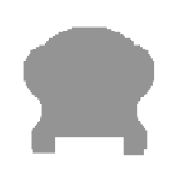
# Autodesk Inventor part: Поручень
Saved by Autodesk Inventor 2019 (Build 230136000, 136)
## iProperties
_CCFamilyDisplayName: Поручень - Ограждение
_FrameMemberDoc: Frame Member File
_Version: 15.0.0
_GetPNFromCC: 1
Created: 2018-10-11
Part Number: Поручень
Material: Древесина (дуб)
Description: Ограждение
Document SubType Name: Modeling
Standard: Без имени
Designer: Андреев Н.Л.
Language: ru-RU
Size Designation: Поручень x75 x58
Categories: <MemberInstance><Categories><Category DisplayName="Профили фасонные" InternalName="089c4875-fa83-4c05-b084-43b9cc11f5ed" Mnemonic="GRDR"><CategoryParameter DisplayName="Вес погонного метра" InternalName="0bb95a10-148f-4027-a459-38d7b056702a" Mnemonic="shpmass"/><CategoryParameter DisplayName="Площадь сечения" InternalName="1ff91680-64b0-4202-b9a3-7fd3f94bba3b" Mnemonic="secarea"/><CategoryParameter DisplayName="Радиус инерции (x)" InternalName="25778675-03e9-40c1-b6a8-4a9ed693320d" Mnemonic="gyrradx"/><CategoryParameter DisplayName="Модуль жесткости при кручении" InternalName="26c1ec35-5026-4c63-ad0a-751cf684a536" Mnemonic="torrigmod"/><CategoryParameter DisplayName="Расстояние центра тяжести X-X" InternalName="26c9bdb8-9c79-4b4f-a92e-8e197583c9c4" Mnemonic="grcendistX"/><CategoryParameter DisplayName="Старое обозначение элемента" InternalName="340afe4f-75d7-48d3-ab7d-943f3c3da468" Mnemonic="LegacyMemberID"/><CategoryParameter DisplayName="Основная длина" InternalName="42e34263-8f20-4d0e-ad48-bf1385b87c24" Mnemonic="shplen"/><CategoryParameter DisplayName="Момент инерции (y)" InternalName="4b9f58ea-bced-460e-81ea-3d29ca5a49e3" Mnemonic="inermomy"/><CategoryParameter DisplayName="Момент инерции (x)" InternalName="4cd780bc-73d7-43ac-917a-579e5cbd684d" Mnemonic="inermomx"/><CategoryParameter DisplayName="Настраиваемые базовые точки" InternalName="4f1d1b73-316d-484b-a3df-9cbabb16eb77" Mnemonic="shpBasePoint"/><CategoryParameter DisplayName="Высота фигуры" InternalName="50274e7d-5ac0-4796-92cb-c59e54983c67" Mnemonic="shpheig"/><CategoryParameter DisplayName="Момент сопротивления сечения (y)" InternalName="59eaa5e9-d227-48dc-b6c1-6920f96e0f95" Mnemonic="secmody"/><CategoryParameter DisplayName="Обозначение разреза" InternalName="5a64d034-428d-49c8-ba32-7619764de20f" Mnemonic="shpdes"/><CategoryParameter DisplayName="Момент сопротивления сечения (x)" InternalName="72cfad18-cf51-4ed4-aaa7-c6b224f8419f" Mnemonic="secmodx"/><CategoryParameter DisplayName="Торсионный момент сопротивления сечения" InternalName="7c55a8dc-8844-49f9-a867-cc677b30ec9a" Mnemonic="torsecmod"/><CategoryParameter DisplayName="Ширина фигуры" InternalName="7c717d54-a18f-4666-b4d4-573cce22c62c" Mnemonic="shpwdth"/><CategoryParameter DisplayName="Толщина второй фигуры" InternalName="9251a8e1-85fd-4e47-af99-afdb762317d9" Mnemonic="shpthick2"/><CategoryParameter DisplayName="Созданные с помощью генератора рам" InternalName="9c666724-f362-4ea7-ac62-f6a007de5c69" Mnemonic="shpFGAuto"/><CategoryParameter DisplayName="Расстояние центра тяжести Y-Y" InternalName="bcc4fb17-7af4-436a-8f8c-d0aa3b0248c5" Mnemonic="grcendistY"/><CategoryParameter DisplayName="Радиус инерции (y)" InternalName="bfa18ebe-1636-4dbe-8d42-b263e0b73184" Mnemonic="gyrrady"/><CategoryParameter DisplayName="Толщина фигуры" InternalName="d109cf76-8eb4-42fc-9800-4409734adc67" Mnemonic="shpthick"/><CategoryParameter DisplayName="Коэффициент смещения при сдвиге" InternalName="de4c90c6-aaa8-468f-a335-6737b311b5d3" Mnemonic="shdispc"/><Category DisplayName="Специальные" InternalName="f02205ff-2390-476f-921c-0b3185f88e84" Mnemonic="OTHSHP"><CategoryParameter DisplayName="Момент инерции (y)" InternalName="044c654e-f649-48ac-84cc-650a29ae31ca" Mnemonic="inermomy"/><CategoryParameter DisplayName="Толщина фигуры" InternalName="12b1a788-9233-48fd-a933-2df8ff42b15f" Mnemonic="shpthick"/><CategoryParameter DisplayName="Вес погонного метра" InternalName="2fd289d6-9394-4d2d-97e6-6659d7d4551d" Mnemonic="shpmass"/><CategoryParameter DisplayName="Радиус инерции (y)" InternalName="743e1dfe-1bba-408b-b985-cf752b207386" Mnemonic="gyrrady"/><CategoryParameter DisplayName="Момент сопротивления сечения (y)" InternalName="88b8bff9-a616-4028-93d5-ed4f79680d13" Mnemonic="secmody"/><CategoryParameter DisplayName="Площадь сечения" InternalName="c46ecdf8-b6eb-4db9-8b25-30258930c1e3" Mnemonic="secarea"/><CategoryParameter DisplayName="Момент сопротивления сечения (x)" InternalName="cac70804-9d39-43bb-be17-56ea1f39a6c2" Mnemonic="secmodx"/><CategoryParameter DisplayName="Момент инерции (x)" InternalName="ec6737bc-264f-43ed-b0bd-f6d410c2718d" Mnemonic="inermomx"/><CategoryParameter DisplayName="Радиус инерции (x)" InternalName="ee72c61e-565e-4fd6-b448-66e1e1abcb7e" Mnemonic="gyrradx"/></Category></Category><Category DisplayName="ТипДанных" InternalName="23b78d0f-2648-40c6-8793-ca6db495c9e8" Mnemonic="DATATYPE"><CategoryParameter DisplayName="ОтображаемоеИмя" InternalName="05415f3d-3907-474b-a020-eb9d644f4cf3" Mnemonic="DISPLAYNAME"/><CategoryParameter DisplayName="Стандарт" InternalName="0c0a119c-1e12-4c84-803f-101930972f5e" Mnemonic="STANDARD"/><CategoryParameter DisplayName="Наименование" InternalName="13903e3d-64b1-4950-80da-f627842ea37f" Mnemonic="DESCRIPTION"/><CategoryParameter DisplayName="Обозначение" InternalName="2675968c-4ce5-49e0-a4f5-552d29089031" Mnemonic="DESIGNATION"/><CategoryParameter DisplayName="Строка по умолчанию" InternalName="2af9ec52-faaa-4026-b378-f9fa4afca842" Mnemonic="DEFAULTROW"/><CategoryParameter DisplayName="Имя папки" InternalName="3f06958e-8713-4116-9be7-ed6184ecc97b" Mnemonic="FOLDERNAME"/><CategoryParameter DisplayName="Указатель редакций" InternalName="45a75005-10b1-4dfc-8d6d-dfe629f0b93c" Mnemonic="REVISIONGUID"/><CategoryParameter DisplayName="ИмяФайла" InternalName="8b46a4cc-9585-4fed-90c3-899f57e09a73" Mnemonic="FILENAME"/><CategoryParameter DisplayName="ОргСтанд" InternalName="8f5914e1-4693-403f-8ab5-d37768198c9d" Mnemonic="STDSORG"/><CategoryParameter DisplayName="Версия семейства" InternalName="914462f6-6e19-4b14-ba84-155b9680b1d0" Mnemonic="FAMILYREVISION"/><CategoryParameter DisplayName="Редакция стандарта" InternalName="91d5a463-65c2-4fde-b823-3b7fea5e8e17" Mnemonic="STANDARDREVISION"/><CategoryParameter DisplayName="редакция элемента" InternalName="a65d44b9-392f-4f4f-857b-e4b3d54996fe" Mnemonic="MEMBERREVISION"/><CategoryParameter DisplayName="ФорматКлипа" InternalName="bc51e27b-3422-4e78-93ef-cec197ddf230" Mnemonic="CLIPFORMAT"/><CategoryParameter DisplayName="Изготовитель" InternalName="cd6c7a72-a28a-4e50-99a9-2c7f4e13e5ad" Mnemonic="MANUFACTURER"/><CategoryParameter DisplayName="ВнутреннееИмя" InternalName="cf1d0246-76d9-4b4a-8305-fa0409afb5c1" Mnemonic="INTERNALNAME"/><CategoryParameter DisplayName="Метрическая" InternalName="e2385c5b-1ea4-4823-96a8-8de651266ec3" Mnemonic="ISMETRIC"/><Category DisplayName="Деталь" InternalName="c0e0b642-3bcb-4cc8-9e80-f96d35c4afa4" Mnemonic="PART"><CategoryParameter DisplayName="Номер детали" InternalName="016b6077-bfbe-49bd-92c9-d8d59c39c941" Mnemonic="PARTNUMBER"/><CategoryParameter DisplayName="Инвентарный номер" InternalName="4dba7c1c-e26c-444e-836c-b08b433409a8" Mnemonic="STOCKNUMBER"/><CategoryParameter DisplayName="Ключ материала" InternalName="5c9a8adb-dd2b-4535-b97f-0a94a95fe41f" Mnemonic="MATERIALKEY"/><CategoryParameter DisplayName="Материал" InternalName="818a152a-d3c3-49ca-80ee-df7d91421b8e" Mnemonic="MATERIAL"/></Category></Category></Categories><FamilyTemplate Id="Поручень"><FamilyTemplateParameters><FamilyTemplateParameter ObjectType="kModelParameterObject" ValueType="xs:double" Id="12" ObjectReferenceKey="ДЛИНА"/><FamilyTemplateParameter ObjectType="kUserParameterObject" ValueType="xs:double" Id="13" ObjectReferenceKey="ШИРИНА"/><FamilyTemplateParameter ObjectType="kUserParameterObject" ValueType="xs:double" Id="14" ObjectReferenceKey="ТОЛЩВЫС"/><FamilyTemplateParameter ObjectType="kPartComponentDefinitionObject" ValueType="xs:string" Id="25" SubObjectId="Material"/><FamilyTemplateParameter ObjectType="kPropertyObject" ValueType="xs:string" Id="27" ObjectReferenceKey="{32853F0F-3444-11d1-9E93-0060B03C1CA6}" SubObjectId="5"/><FamilyTemplateParameter ObjectType="kPropertyObject" ValueType="xs:string" Id="28" ObjectReferenceKey="{32853F0F-3444-11d1-9E93-0060B03C1CA6}" SubObjectId="52"/></FamilyTemplateParameters></FamilyTemplate><CategoryParameterMap><ParamToTemplateMap><ParamToTemplate CategoryParameter="//CategoryParameter[@InternalName='cf1d0246-76d9-4b4a-8305-fa0409afb5c1']" ConstantValue="9f81204e-1447-4a53-895e-ded6cb6d2cf7"/><ParamToTemplate CategoryParameter="//CategoryParameter[@InternalName='45a75005-10b1-4dfc-8d6d-dfe629f0b93c']" ConstantValue="d7f6d775-39c0-4cd3-8369-c535a5b7ca87"/><ParamToTemplate CategoryParameter="//CategoryParameter[@InternalName='3f06958e-8713-4116-9be7-ed6184ecc97b']" ConstantValue="Поручень"/><ParamToTemplate CategoryParameter="//CategoryParameter[@InternalName='8f5914e1-4693-403f-8ab5-d37768198c9d']" TemplateParameter="19"/><ParamToTemplate CategoryParameter="//CategoryParameter[@InternalName='0c0a119c-1e12-4c84-803f-101930972f5e']" TemplateParameter="20"/><ParamToTemplate CategoryParameter="//CategoryParameter[@InternalName='91d5a463-65c2-4fde-b823-3b7fea5e8e17']" TemplateParameter="21"/><ParamToTemplate CategoryParameter="//CategoryParameter[@InternalName='cd6c7a72-a28a-4e50-99a9-2c7f4e13e5ad']" TemplateParameter="22"/><ParamToTemplate CategoryParameter="//CategoryParameter[@InternalName='13903e3d-64b1-4950-80da-f627842ea37f']" ConstantValue="Ограждение"/><ParamToTemplate CategoryParameter="//CategoryParameter[@InternalName='05415f3d-3907-474b-a020-eb9d644f4cf3']" ConstantValue="Поручень"/><ParamToTemplate CategoryParameter="//CategoryParameter[@InternalName='914462f6-6e19-4b14-ba84-155b9680b1d0']" ConstantValue="11"/><ParamToTemplate CategoryParameter="//CategoryParameter[@InternalName='bc51e27b-3422-4e78-93ef-cec197ddf230']" ConstantValue="CF_INVENTOR.STDPARTS"/><ParamToTemplate CategoryParameter="//CategoryParameter[@InternalName='e2385c5b-1ea4-4823-96a8-8de651266ec3']" ConstantValue="true"/><ParamToTemplate CategoryParameter="//CategoryParameter[@InternalName='2af9ec52-faaa-4026-b378-f9fa4afca842']" ConstantValue="1"/><ParamToTemplate CategoryParameter="//CategoryParameter[@InternalName='4f1d1b73-316d-484b-a3df-9cbabb16eb77']" ConstantValue="1"/><ParamToTemplate CategoryParameter="//CategoryParameter[@InternalName='9c666724-f362-4ea7-ac62-f6a007de5c69']" ConstantValue="1"/><ParamToTemplate CategoryParameter="//CategoryParameter[@InternalName='8b46a4cc-9585-4fed-90c3-899f57e09a73']" ConstantValue="Поручень-75-58-10"/><ParamToTemplate CategoryParameter="//CategoryParameter[@InternalName='a65d44b9-392f-4f4f-857b-e4b3d54996fe']" ConstantValue="856d8d5c-2c60-46fb-910a-dbf8e98beac2"/><ParamToTemplate CategoryParameter="//CategoryParameter[@InternalName='a65d44b9-392f-4f4f-857b-e4b3d54996fe']" ConstantValue="856d8d5c-2c60-46fb-910a-dbf8e98beac2"/><ParamToTemplate CategoryParameter="//CategoryParameter[@InternalName='2675968c-4ce5-49e0-a4f5-552d29089031']" TemplateParameter="28"/><ParamToTemplate CategoryParameter="//CategoryParameter[@InternalName='818a152a-d3c3-49ca-80ee-df7d91421b8e']" TemplateParameter="25"/><ParamToTemplate CategoryParameter="//CategoryParameter[@InternalName='016b6077-bfbe-49bd-92c9-d8d59c39c941']" TemplateParameter="27"/><ParamToTemplate CategoryParameter="//CategoryParameter[@InternalName='42e34263-8f20-4d0e-ad48-bf1385b87c24']" TemplateParameter="12"/><ParamToTemplate CategoryParameter="//CategoryParameter[@InternalName='12b1a788-9233-48fd-a933-2df8ff42b15f']" TemplateParameter="14"/><ParamToTemplate CategoryParameter="//CategoryParameter[@InternalName='7c717d54-a18f-4666-b4d4-573cce22c62c']" TemplateParameter="13"/></ParamToTemplateMap></CategoryParameterMap></MemberInstance>
Density: 0.76 g/cm^3
Appearance: Белый дуб — натуральный — с умеренным глянцем
Mass: 8224.83 g
Surface Area: 8964.03 cm^2
Volume: 10822.1 cm^3
IsCustomPart: 1
ШИРИНА: 75
ТОЛЩВЫС: 58
ДЛИНА: 1691,866 мм
G_L: 3449,661 мм
G_W: 73,967 мм
G_H: 57,530 мм
+5CDBFC76-318E-43F1-8F52-CB9B587A4B74+ВЫНОСНОЙЭЛЕМЕНТ1: Угол среза 61,30 град
+F6280B44-C2CE-4FF6-9F4F-F8700B51F05E+ВЫНОСНОЙЭЛЕМЕНТ2: Угол среза 61,30 град
Author: Андреев Н.Л.
Autodesk Inventor part; units mm, degrees
sketch "Поручень" plane through (0, 0, 0) normal (0, 0, 1) x (1, 0, 0)
  line L0 (20.3655, -7.6059) -> (20.3655, -0.2092)
  line L1 (20.3655, -0.2092) -> (-19.6345, -0.2092)
  line L2 (-19.6345, -0.2092) -> (-19.6345, -7.6059)
  line L3 (-19.6345, -7.6059) -> (-30.865, -7.6059)
  line L4 (-30.865, -7.6059) -> (-30.865, -5.9622)
  line L5 (-30.865, -5.9622) -> (-32.5087, -5.9622)
  line L6 (-32.5087, -5.9622) -> (-32.5087, 0.6126)
  arc A0 (-30.367, 4.2203) -> (-32.5087, 0.6126) centre (-28.3995, 0.6126) ccw
  arc A1 (-30.367, 4.2203) -> (-30.2973, 18.6123) centre (-34.302, 11.4355) ccw
  arc A2 (-24.2902, 41.7054) -> (-30.2973, 18.6123) centre (-24.2902, 29.3776) ccw
  line L7 (-24.2902, 41.7054) -> (-24.2902, 42.9382)
  arc A3 (25.0211, 42.9382) -> (-24.2902, 42.9382) centre (0.3655, 2.9211) ccw
  line L8 (25.0211, 42.9382) -> (25.0211, 41.7054)
  arc A4 (31.0282, 18.6123) -> (25.0211, 41.7054) centre (25.0211, 29.3776) ccw
  arc A5 (31.0282, 18.6123) -> (31.0979, 4.2203) centre (35.033, 11.4355) ccw
  arc A6 (33.2397, 0.6126) -> (31.0979, 4.2203) centre (29.1304, 0.6126) ccw
  line L9 (33.2397, 0.6126) -> (33.2397, -5.9622)
  line L10 (33.2397, -5.9622) -> (31.596, -5.9622)
  line L11 (31.596, -5.9622) -> (31.596, -7.6059)
  line L12 (31.596, -7.6059) -> (20.3655, -7.6059)
  point P0 (0.3655, -0.2092)
  point P1 (0.3655, -7.6059)
sketch "Эскиз" plane through (0, 0, 0) normal (0, 0, 1) x (1, 0, 0)
  line L0 (20, 0) -> (20, 7.3967)
  line L1 (20, 7.3967) -> (-20, 7.3967)
  line L2 (-20, 7.3967) -> (-20, 0)
  line L3 (-20, 0) -> (-31.2305, 0)
  line L4 (-31.2305, 0) -> (-31.2305, 1.6437)
  line L5 (-31.2305, 1.6437) -> (-32.8742, 1.6437)
  line L6 (-32.8742, 1.6437) -> (-32.8742, 8.2186)
  arc A0 (-30.7325, 11.8262) -> (-32.8742, 8.2186) centre (-28.7649, 8.2186) ccw
  arc A1 (-30.7325, 11.8262) -> (-30.6628, 26.2183) centre (-34.6675, 19.0415) ccw
  arc A2 (-24.6557, 49.3113) -> (-30.6628, 26.2183) centre (-24.6557, 36.9835) ccw
  line L7 (-24.6557, 49.3113) -> (-24.6557, 50.5441)
  arc A3 (24.6557, 50.5441) -> (-24.6557, 50.5441) centre (0, 10.527) ccw
  line L8 (24.6557, 50.5441) -> (24.6557, 49.3113)
  arc A4 (30.6628, 26.2183) -> (24.6557, 49.3113) centre (24.6557, 36.9835) ccw
  arc A5 (30.6628, 26.2183) -> (30.7325, 11.8262) centre (34.6675, 19.0415) ccw
  arc A6 (32.8742, 8.2186) -> (30.7325, 11.8262) centre (28.7649, 8.2186) ccw
  line L9 (32.8742, 8.2186) -> (32.8742, 1.6437)
  line L10 (32.8742, 1.6437) -> (31.2305, 1.6437)
  line L11 (31.2305, 1.6437) -> (31.2305, 0)
  line L12 (31.2305, 0) -> (20, 0)
  point P0 (0, 0)
  constraints: 1 other
ref_plane "Начальная плоскость" through (0, 0, -756.0582) normal (0, 0, 1) x (1, 0, 0)
ref_plane "РабПлоскость2" through (0, 0, 1691.8665) normal (0, 0, 1) x (1, 0, 0)
extrude "Тело" add sketch "Эскиз" along normal up to surface (3449.6612 mm away) from surface at -756.0582
ref_plane "Конечная плоскость" through (0, 0, 2693.603) normal (0, 0, 1) x (1, 0, 0)
ref_plane "РабПлоскость4" through (128.3639, -658.2736, 3054.0122) normal (0, 0.4802388, 0.8771378) x (1, 0, 0)
split "Разделение1" plane through (128.3639, -658.2736, 3054.0122) removes the side toward (0, 0.4802388, 0.8771378)
ref_plane "РабПлоскость5" through (-45, -656.9733, -364.8629) normal (0, -0.4802388, -0.8771378) x (1, 0, 0)
split "Разделение2" plane through (-45, -656.9733, -364.8629) removes the side toward (0, -0.4802388, -0.8771378)
equation "\"ШИРИНА\" = 75"
equation "\"ТОЛЩВЫС\" = 58"
equation "\"d0\" = -G_OFFSET_START"
equation "\"СЕЧЕНИЕ_СМЕЩ\" = 0"
equation "\"G_OFFSET_END\" = 1001.73648"
equation "\"d4\" = ДЛИНА + G_OFFSET_END"
equation "\"G_OFFSET_START\" = 756.05818"
equation "\"G_L\" = ДЛИНА + G_OFFSET_START + G_OFFSET_END"
equation "\"ДЛИНА\" = 1691.866499"
